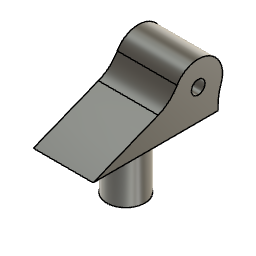
Ankle v1 (Autodesk Fusion 360 archive; units mm, degrees)
design "Spring Peg"
Autodesk Fusion 360 part; units mm, degrees
sketch "Sketch1" plane through (0, 0, 0) normal (0, 0, 1) x (1, 0, 0)
sketch "Sketch2" plane through (0, 0, 0) normal (1, 0, 0) x (0, 1, 0)
  line L0 (0, 0) -> (23, 0)
  line L1 (0, 0) -> (14.8556, 5.9423)
  line L2 (23, 0) -> (29.4822, 0) construction
  arc A0 (23, 3) -> (14.8556, 5.9423) centre (19.3245, 5.5692) ccw
  circle A1 centre (19.3245, 5.5692) radius 1.25
  line L3 (23, 0) -> (23, 3)
  dimension "d3" = 23
  dimension "d4" = 16
  dimension "d6" = 2.5
  constraint coincident L0.start L1.start
  constraint horizontal L0
  constraint horizontal L2
  constraint concentric A0 A1
  constraint perpendicular L0 L3
  measures "d3" distance of L0.start L0.end
  measures "d4" distance of L0.start L1.end
  measures "d6" diameter of A1
extrude "Extrude1" add sketch "Sketch2" along normal blind 11
fillet "Fillet1" radius 7 1 edges at (5.5, 14.8556, 5.9423)
fillet "Fillet2" radius 8.5 1 edges at (5.5, 23, 3)
sketch "Sketch3" plane through (0, 0, 0) normal (0, 0, -1) x (1, 0, 0)
  line L0 (0, 0) -> (0, -23)
  line L1 (0, -23) -> (11, -23)
  line L2 (11, -23) -> (11, 0)
  line L3 (11, 0) -> (0, 0)
  circle A0 centre (5.5, -11.5) radius 3.5
  dimension "d13" = 7
  measures "d13" diameter of A0
extrude "Extrude2" add sketch "Sketch3" along normal blind 10 contours A0

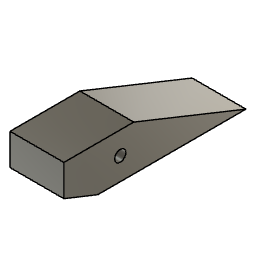
design "Forefoot peg"
Autodesk Fusion 360 part; units mm, degrees
sketch "Sketch1" plane through (0, 0, 0) normal (1, 0, 0) x (0, 1, 0)
  line L0 (0, 0) -> (33, 0)
  line L1 (33, 0) -> (8, 10)
  line L2 (33, 0) -> (38.0278, 0) construction
  line L3 (8, 10) -> (-7.5578, 10)
  line L4 (-7.5578, 10) -> (-7.5578, 3)
  line L5 (-7.5578, 3) -> (0, 0)
  line L6 (5, 0) -> (5, 5)
  circle A0 centre (5, 5) radius 1.25
  dimension "d4" = 7
  dimension "d5" = 2.5
  constraint coincident L0.start L5.end
  constraint horizontal L0
  constraint horizontal L2
  constraint horizontal L3
  constraint perpendicular L3 L4
  constraint coincident L0 L6.start
  constraint perpendicular L0 L6
  constraint coincident L6.end A0.centre
  measures "d4" distance of L3.end L4.end
  measures "d5" diameter of A0
extrude "Extrude1" add sketch "Sketch1" along normal blind 12
sketch "Sketch2" plane through (0, 4.5517, 11.3793) normal (0, 0.371391, 0.928477) x (-1, 0, 0)
  line L0 (0, -30.6397) -> (0, -3.7139)
  line L1 (0, -3.7139) -> (-12, -3.7139)
  line L2 (-12, -3.7139) -> (-12, -30.6397)
  line L3 (-12, -30.6397) -> (0, -30.6397)
  circle A0 centre (-6, -3) radius 2
sketch "Sketch3" plane through (0, 0, 0) normal (0, 0, -1) x (1, 0, 0)
  line L0 (0, 0) -> (0, -33)
  line L1 (0, -33) -> (12, -33)
  line L2 (12, -33) -> (12, 0)
  line L3 (12, 0) -> (0, 0)
  circle A0 centre (6, -30) radius 2
  dimension "d10" = 4
  measures "d10" diameter of A0
extrude "Extrude3" add sketch "Sketch3" along normal blind 3 contours A0
